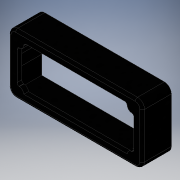
# Autodesk Inventor part: EC3BK-40mm_Case_EndCap
Saved by Autodesk Inventor 2016 (Build 200138000, 138)
## iProperties
Created: 2016-09-24
Part Number: EC3BK-40mm_Case_EndCap
Material: Generic
Document SubType Name: Modeling
Designer: jfixelle
Density: 1 g/cm^3
Appearance: Black
Author: jfixelle
Autodesk Inventor part; units mm, degrees
ref_plane "YZ Plane" through (0, 0, 0) normal (1, 0, 0) x (0, 1, 0)
ref_plane "XZ Plane" through (0, 0, 0) normal (0, 1, 0) x (-1, 0, 0)
ref_plane "XY Plane" through (0, 0, 0) normal (0, 0, 1) x (1, 0, 0)
sketch "Sketch1" plane through (0, 0, 0) normal (0, 0, 1) x (1, 0, 0)
  line L0 (-57.23, 25.5) -> (57.23, 25.5)
  line L1 (57.23, 25.5) -> (57.23, -25.48)
  line L2 (57.23, -25.48) -> (-57.23, -25.48)
  line L3 (-57.23, -25.48) -> (-57.23, 25.5)
  line L4 (-42.25, 19) -> (42.25, 19)
  line L5 (50, 11.3) -> (50, -13.2)
  line L6 (-50, -13.2) -> (-50, 11.3)
  line L7 (-53.6456, 17.3) -> (53.2492, 17.3) construction
  line L8 (-53.6456, -19.2) -> (53.2492, -19.2) construction
  line L9 (48.25, -31.9957) -> (48.25, 43.3545) construction
  line L10 (-48.25, 39.0692) -> (-48.25, -34.8525) construction
  line L11 (48.25, -15.2) -> (48, -15.2)
  line L12 (48.25, 13.3) -> (48, 13.3)
  line L13 (44.25, 17.3) -> (44.25, 17)
  line L14 (-48.25, 13.3) -> (-48, 13.3)
  line L15 (-44.25, 17.3) -> (-44.25, 17)
  line L16 (-48.25, -15.2) -> (-48, -15.2)
  arc A0 (-50, -13.2) -> (-48, -15.2) centre (-48, -13.2) ccw
  arc A1 (-48, 13.3) -> (-50, 11.3) centre (-48, 11.3) ccw
  arc A2 (-42.25, 19) -> (-44.25, 17) centre (-42.25, 17) ccw
  arc A3 (44.25, 17) -> (42.25, 19) centre (42.25, 17) ccw
  arc A4 (50, 11.3) -> (48, 13.3) centre (48, 11.3) ccw
  arc A5 (48, -15.2) -> (50, -13.2) centre (48, -13.2) ccw
  arc A6 (52.25, 17.3) -> (48.25, 21.3) centre (48.25, 17.3) ccw
  arc A7 (44.25, 17.3) -> (48.25, 13.3) centre (48.25, 17.3) ccw
  arc A8 (48.25, -15.2) -> (44.25, -19.2) centre (48.25, -19.2) ccw
  arc A9 (48.25, -23.2) -> (52.25, -19.2) centre (48.25, -19.2) ccw
  line L17 (50, -19) -> (48.25, -19)
  arc A10 (-48.25, 13.3) -> (-44.25, 17.3) centre (-48.25, 17.3) ccw
  arc A11 (-48.25, 21.3) -> (-52.25, 17.3) centre (-48.25, 17.3) ccw
  arc A12 (-44.25, -19.2) -> (-48.25, -15.2) centre (-48.25, -19.2) ccw
  arc A13 (-52.25, -19.2) -> (-48.25, -23.2) centre (-48.25, -19.2) ccw
  line L18 (44.255, -19) -> (-44.255, -19)
  line L19 (-48.25, -19) -> (-50, -19)
  point P0 (0, 0)
  point P1 (-50, 19)
  point P2 (50, 19)
  point P3 (-50, 13.3)
  point P4 (-50, -15.2)
  dimension "d0" = 114.46
  dimension "d1" = 57.23
  dimension "d2" = 25.5
  dimension "d3" = 25.48
  dimension "d4" = 100
  dimension "d10" = 50
  dimension "d11" = 17.3
  dimension "d12" = 19.2
  dimension "d13" = 96.5
  dimension "d14" = 48.25
  dimension "d19" = 2
  dimension "d20" = 2
  constraints: 38 end point, 31 point on line, 30 point on circle, 16 tangent, 14 centre point, 7 perpendicular, 6 parallel, 4 equal radius, 3 horizontal, 1 vertical, 10 other
  measures "d0" distance of L0.start L0.end
  measures "d1" distance from line of point (0, 0) L1
  measures "d2" distance from line of point (0, 0) L0
  measures "d3" distance from line of point (0, 0) L2
  measures "d4" distance of point (-50, 19) point (50, 19)
  measures "d10" distance from line of L5 point (0, 0)
  measures "d11" distance from line of point (0, 0) L7
  measures "d12" distance from line of L8 point (0, 0)
  measures "d14" distance from line of point (0, 0) L10
  measures "d19" radius of A0
  measures "d20" radius of A1
extrude "Extrusion1" add sketch "Sketch1" along normal blind 4
sketch "Sketch2" plane through (0, 0, 0) normal (0, 0, -1) x (-1, 0, 0)
  line L0 (57.23, -25.48) -> (57.23, 25.5) projected
  line L1 (57.23, -25.48) -> (-57.23, -25.48) projected
  line L2 (57.23, 25.5) -> (-57.23, 25.5)
  line L3 (-57.23, 25.5) -> (-57.23, -25.48)
  line L4 (-57.23, -25.48) -> (57.23, -25.48)
  line L5 (57.23, -25.48) -> (57.23, 25.5)
  line L6 (53.885, 22.255) -> (-53.885, 22.255)
  line L7 (-53.885, 22.255) -> (-53.885, -22.255)
  line L8 (-53.885, -22.255) -> (53.885, -22.255)
  line L9 (53.885, -22.255) -> (53.885, 22.255)
  line L10 (-53.885, 5.805) -> (-51.735, 5.805)
  line L11 (-51.735, 5.805) -> (-51.735, -5.805)
  line L12 (-51.735, -5.805) -> (-53.885, -5.805)
  line L13 (-53.885, -5.805) -> (-53.885, 5.805)
  line L14 (53.885, 5.805) -> (51.735, 5.805)
  line L15 (51.735, 5.805) -> (51.735, -5.805)
  line L16 (51.735, -5.805) -> (53.885, -5.805)
  line L17 (53.885, -5.805) -> (53.885, 5.805)
  line L18 (-51.735, 4.5637) -> (-53.885, 5.805)
  line L19 (-51.735, -4.5637) -> (-53.885, -5.805)
  line L20 (51.735, 4.5637) -> (53.885, 5.805)
  line L21 (51.735, -4.5637) -> (53.885, -5.805)
  point P0 (0, 0)
  dimension "d23" = 44.51
  dimension "d24" = 22.255
  dimension "d25" = 107.77
  dimension "d26" = 53.885
  dimension "d28" = 103.47
  dimension "d30" = 51.735
  dimension "d31" = 11.61
  dimension "d32" = 5.805
  dimension "d33" = 11.61
  dimension "d34" = 5.805
  dimension "d35" = 30
  dimension "d36" = 30
  dimension "d37" = 30
  dimension "d38" = 30
  constraints: 40 end point, 8 parallel, 6 point on line, 4 horizontal, 4 perpendicular
  measures "d23" distance of L6.end L7.end
  measures "d24" distance from line of point (0, 0) L8
  measures "d25" distance of L7.end L8.end
  measures "d26" distance from line of point (0, 0) L7
  measures "d28" distance between parallel lines of L15 L11
  measures "d30" distance from line of L15 point (0, 0)
  measures "d31" distance of L14.end L15.end
  measures "d32" distance from line of point (0, 0) L14
  measures "d33" distance of L10.end L11.end
  measures "d34" distance from line of point (0, 0) L10
  measures "d35" angle of L16 L21
  measures "d36" angle of L14 L20
  measures "d37" angle of L12 L19
  measures "d38" angle of L10 L18
extrude "Extrusion2" add sketch "Sketch2" along normal blind 21 contours L1 L3 L2 L0 | L9 L21 L15 L20 | L18 L11 L19 L7
fillet "Fillet1" radius 6 4 edges at (57.23, 25.5, -8.5) (-57.23, 25.5, -8.5) (57.23, -25.48, -8.5) (-57.23, -25.48, -8.5)
fillet "Fillet2" radius 2 8 edges at (0, -25.48, 4) (55.4726, -23.7226, 4) (57.23, 0.01, 4) (55.4726, 23.7426, 4) (0, 25.5, 4) (-55.4726, 23.7426, 4) (-57.23, 0.01, 4) (-55.4726, -23.7226, 4)
body "Solid1"
